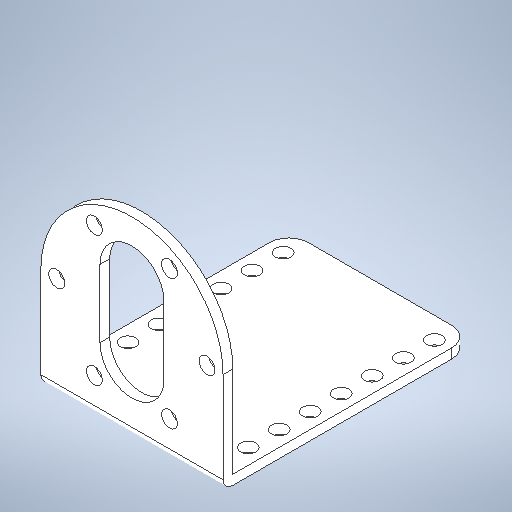
# Autodesk Inventor part: L-Bracket
Saved by Autodesk Inventor 2026.2 (Build 302298010, 298A)
## iProperties
Created: 2026-05-06
Part Number: L-Bracket
Material: 一般
Document SubType Name: Modeling
Designer: Yagis
Density: 1 g/cm^3
Appearance: 既定
Author: Yagis
Autodesk Inventor part; units mm, degrees
ref_plane "YZ Plane" through (0, 0, 0) normal (1, 0, 0) x (0, 1, 0)
ref_plane "XZ Plane" through (0, 0, 0) normal (0, 1, 0) x (-1, 0, 0)
ref_plane "XY Plane" through (0, 0, 0) normal (0, 0, 1) x (1, 0, 0)
sketch "スケッチ1" plane through (0, 0, 0) normal (0, 0, 1) x (1, 0, 0)
  line L0 (0, 0) -> (37.6, 0)
  line L1 (37.6, 0) -> (37.6, 20.8)
  line L2 (37.6, 20.8) -> (0, 20.8)
  line L3 (0, 20.8) -> (0, 0)
  line L4 (0, 2) -> (37.6, 2)
  arc A0 (37.6, 20.8) -> (0, 20.8) centre (18.8, 20.8) ccw
  line L5 (12.2, 27.8) -> (25.4, 27.8)
  line L6 (25.4, 27.8) -> (25.4, 13.8)
  line L7 (25.4, 13.8) -> (12.2, 13.8)
  line L8 (12.2, 13.8) -> (12.2, 27.8)
  arc A1 (25.4, 27.8) -> (12.2, 27.8) centre (18.8, 27.8) ccw
  arc A2 (12.2, 13.8) -> (25.4, 13.8) centre (18.8, 13.8) ccw
  point P0 (18.8, 20.8)
  point P1 (18.8, 39.6)
  dimension "d0" = 37.6
  dimension "d1" = 20.8
  dimension "d2" = 2
  dimension "d3" = 18.8
  dimension "d4" = 13.2
  dimension "d5" = 14
  dimension "d6" = 7
  dimension "d7" = 18.8
  constraints: 18 end point, 7 point on circle, 4 parallel, 4 tangent, 3 centre point, 3 perpendicular, 2 horizontal, 2 midpoint, 2 point on line
  measures "d0" distance of L0.start L0.end
  measures "d1" distance of L2.end L0.start
  measures "d2" distance between parallel lines of L0 L4
  measures "d3" distance of point (18.8, 20.8) point (18.8, 39.6)
  measures "d4" distance between parallel lines of L8 L6
  measures "d5" distance between parallel lines of L7 L5
  measures "d6" distance between parallel lines of L2 L7
  measures "d7" distance from line of L1 point (18.8, 13.8)
extrude "押し出し1" add sketch "スケッチ1" against normal blind 2 contours L3 L2 L8 A2 L6 L1 L4 | A0 L2 L6 A1 L8
extrude "押し出し2" add sketch "スケッチ1" against normal blind 51.2 contours L3 L4 L1 L0
sketch "スケッチ2" plane through (0, 0, 0) normal (0, 0, 1) x (1, 0, 0)
  line L0 (0, 0) -> (37.6, 0) projected
  line L1 (0, 20.8) -> (0, 0) projected
  point P0 (3.3, 20.8)
  point P1 (18.8, 20.8)
  point P2 (11.05, 7.3766)
  point P3 (26.55, 7.3766)
  point P4 (34.3, 20.8)
  point P5 (26.55, 34.2234)
  point P6 (11.05, 34.2234)
  dimension "d12" = 20.8
  dimension "d13" = 18.8
  dimension "d16" = 360
  dimension "d18" = 15.5
  constraints: 1 horizontal alignment, 7 other
  measures "d12" distance from line of L0 point (3.3, 20.8)
  measures "d13" distance from line of L1 point (18.8, 20.8)
  measures "d18" distance of point (3.3, 20.8) point (18.8, 20.8)
hole "穴1" at (3.3, 20.8, 0) at (18.8, 20.8, 0) at (11.05, 7.3766, 0) at (26.55, 7.3766, 0) at (34.3, 20.8, 0) at (26.55, 34.2234, 0) at (11.05, 34.2234, 0) direction (0, 0, -1) diameter 3.3 depth 8.1 tip angle 118
sketch "スケッチ3" plane through (0, 2, -2) normal (0, 1, 0) x (1, 0, 0)
  line L0 (0, -2) -> (37.6, -2) projected
  line L1 (0, 0) -> (0, 49.2) projected
  line L2 (3.2, 6.4) -> (15.917, 6.4)
  line L3 (3.2, 6.4) -> (3.2, 14.7268)
  point P0 (34.4, 6.4)
  point P1 (3.2, 12.8)
  point P2 (34.4, 12.8)
  point P3 (3.2, 19.2)
  point P4 (34.4, 19.2)
  point P5 (3.2, 25.6)
  point P6 (34.4, 25.6)
  point P7 (3.2, 32)
  point P8 (34.4, 32)
  point P9 (3.2, 38.4)
  point P10 (34.4, 38.4)
  point P11 (3.2, 44.8)
  point P12 (34.4, 44.8)
  dimension "d26" = 8.4
  dimension "d27" = 3.2
  dimension "d30" = 31.2
  dimension "d33" = 6.4
  constraints: 4 end point, 2 horizontal, 2 vertical, 13 other
  measures "d26" distance from line of L2.start L0
  measures "d27" distance from line of L2.start L1
  measures "d30" distance of L2.start point (34.4, 6.4)
  measures "d33" distance of L2.start point (3.2, 12.8)
hole "穴2" at (3.2, 2, -8.4) at (34.4, 2, -8.4) at (3.2, 2, -14.8) at (34.4, 2, -14.8) at (3.2, 2, -21.2) at (34.4, 2, -21.2) at (3.2, 2, -27.6) at (34.4, 2, -27.6) at (3.2, 2, -34) at (34.4, 2, -34) at (3.2, 2, -40.4) at (34.4, 2, -40.4) at (3.2, 2, -46.8) at (34.4, 2, -46.8) direction (0, -1, 0) diameter 3.2 depth 8.1 tip angle 118
fillet "面フィレット1" radius 4 1 edges at (37.6, 1, -51.2)
fillet "面フィレット2" radius 4 1 edges at (0, 1, -51.2)
fillet "面フィレット3" radius 2 1 edges at (18.8, 0, 0)
equation "\"d7\" = 0.5 * d0"
